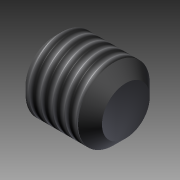
# Autodesk Inventor part: SET-SCREW3-3
Saved by Autodesk Inventor 2011 SP1 (Build 150282100, 282)
## iProperties
Created: 2017-08-06
Part Number: SET-SCREW3-3
Catalog Web Link: www.cadenas.de
Description: SET-SCREW-Set Screw - Flat End
Vendor: MISUMI
Document SubType Name: Modeling
Designer: psAdmin
Manufacturer: MISUMI
Mass: 0.0171527 g
Surface Area: 0.440201 cm^2
Volume: 0.0171527 cm^3
Density: 1 g/cm^3
Category: PARTsolutions
Company: MISUMI
Title: SET-SCREW3-3
Author: Cadenas PARTsolutions
Comments: Set Screw - Flat End
PSOL_IDENT_0: {$CADENAS_DATA\23d-libs\misumi\metric\accessories\set_screw.prj},170 {VTYP=3D},{NB=SET-SCREW3-3},{LI
PSOL_IDENT_1: NA=SET-SCREW3-3},{NN=SET-SCREW},{DATE=17.06.2016 05:56:50},{GEOMDATE=11.12.2013 00:00:00},{VERSION=}
PSOL_IDENT_2: ,{LINEID=30},{LINESUBID=-1},{WBVAR=L}  {NB=SET-SCREW3-3},{LINA=SET-SCREW3-3},{KT=DUMMY},{PN=SET-SCRE
PSOL_IDENT_3: W3-3},{TYPE=SET-SCREW},{M=3.0},{P=0.50},{L=3},{LMIN=1.7},{LALG=[1.7:42/0.1]},{B=1.5},{C=1.2},{DD=2.0
PSOL_IDENT_4: }
NN: SET-SCREW
NT: Set Screw - Flat End
NB: SET-SCREW3-3
NBSYN: $PN.
LINA: SET-SCREW3-3
PN: SET-SCREW3-3
M: 3.0
P: 0.50
L: 3.0
B: 1.5
C: 1.2
DD: 2.0
SUPPLIER: MISUMI
ARTICLENO: SET-SCREW3-3
BOMINFO: SET-SCREW3-3
CREATOR: CADENAS GmbH
Autodesk Inventor part; units mm, degrees
ref_plane "YZ Plane" through (0, 0, 0) normal (1, 0, 0) x (0, 1, 0)
ref_plane "XZ Plane" through (0, 0, 0) normal (0, 1, 0) x (-1, 0, 0)
ref_plane "XY Plane" through (0, 0, 0) normal (0, 0, 1) x (1, 0, 0)
sketch "Sketch_1" plane through (0, 0, 0) normal (0, 0, 1) x (1, 0, 0)
  line L0 (0, 0) -> (-3, 0)
  line L1 (-3, 0) -> (-3, 1.1935)
  line L2 (-3, 1.1935) -> (-2.6935, 1.5)
  line L3 (-2.6935, 1.5) -> (-0.5, 1.5)
  line L4 (-0.5, 1.5) -> (0, 1)
  line L5 (0, 1) -> (0, 0)
  line L6 (0, 0) -> (-3, 0)
  constraints: 14 end point
revolve "Revolution1" add sketch "Sketch_1" angle 360 about axis through (0, 0, 0) along (1, 0, 0)
thread "Thread1" size "M3x0.5" class "6g" standard "ISO Metric profile" full length
sketch "Sketch_2" plane through (-3, 0, 0) normal (-1, 0, 0) x (0, 1, 0)
  line L0 (-0.75, -0.433) -> (0, -0.866)
  line L1 (0, -0.866) -> (0.75, -0.433)
  line L2 (0.75, -0.433) -> (0.75, 0.433)
  line L3 (0.75, 0.433) -> (0, 0.866)
  line L4 (0, 0.866) -> (-0.75, 0.433)
  line L5 (-0.75, 0.433) -> (-0.75, -0.433)
  constraints: 12 end point
extrude "Extrusion1" cut sketch "Sketch_2" against normal blind 1.2
sketch "Sketch_3" plane through (0, 0, 0) normal (0, 0, 1) x (1, 0, 0)
  line L0 (-1.367, 0) -> (-1.8, 0)
  line L1 (-1.8, 0) -> (-1.8, 0.75)
  line L2 (-1.8, 0.75) -> (-1.367, 0)
  line L3 (-1.367, 0) -> (-1.8, 0)
  constraints: 8 end point
revolve "Revolution2" cut sketch "Sketch_3" angle 360 about axis through (-1.367, 0, 0) along (1, 0, 0)
ref_plane "CP_XY" through (0, 0, 0) normal (1, 0, 0) x (0, 0, -1)
ref_plane "CP_YZ" through (0, 0, 0) normal (0, 0, -1) x (0, 1, 0)
ref_plane "CP_ZX" through (0, 0, 0) normal (0, 1, 0) x (1, 0, 0)
body "Solid1"
